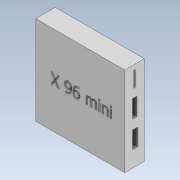
# Autodesk Inventor part: Медиа приставка GIBORIY X96 Mini 2
Saved by Autodesk Inventor 2021.2 (Build 252289000, 289)
## iProperties
Created: 2022-11-29
Part Number: Медиа приставка GIBORIY X96 Mini 2
Material: Типовые
Document SubType Name: Modeling
Designer: Voodoo
Mass: 114.64 g
Surface Area: 238.678 cm^2
Volume: 114.64 cm^3
Density: 1 g/cm^3
Appearance: По умолчанию
Author: Voodoo
Autodesk Inventor part; units mm, degrees
ref_plane "YZ Plane" through (0, 0, 0) normal (1, 0, 0) x (0, 1, 0)
ref_plane "XZ Plane" through (0, 0, 0) normal (0, 1, 0) x (-1, 0, 0)
ref_plane "XY Plane" through (0, 0, 0) normal (0, 0, 1) x (1, 0, 0)
sketch "Эскиз1" plane through (0, 0, 0) normal (0, 0, 1) x (1, 0, 0)
  line L0 (-41, -41) -> (41, -41)
  line L1 (41, -41) -> (41, 41)
  line L2 (41, 41) -> (-41, 41)
  line L3 (-41, 41) -> (-41, -41)
  line L4 (-41, -41) -> (41, 41) construction
  line L5 (41, -41) -> (-41, 41) construction
  point P0 (0, 0)
  dimension "d0" = 82
  dimension "d1" = 82
  constraints: 12 end point, 2 midpoint, 2 parallel, 1 horizontal, 1 perpendicular
  measures "d0" distance of L2.end L1.end
  measures "d1" distance of L1.end L0.end
extrude "Выдавливание1" add sketch "Эскиз1" along normal blind 18
sketch "Эскиз2" plane through (-41, -41, 0) normal (0, -1, 0) x (1, 0, 0)
  line L0 (0, 0) -> (82, 0) projected
  line L1 (82, 0) -> (82, 18) projected
  line L2 (0, 18) -> (82, 18) projected
  line L3 (0, 0) -> (0, 18) projected
  line L4 (21.3532, 13.2427) -> (31.0848, 13.2427)
  line L5 (31.0848, 13.2427) -> (31.0848, 4.7964)
  line L6 (31.0848, 4.7964) -> (21.3532, 4.7964)
  line L7 (21.3532, 4.7964) -> (21.3532, 13.2427)
  line L8 (39.8983, 10.8557) -> (49.9971, 10.8557)
  line L9 (49.9971, 10.8557) -> (49.9971, 6.6326)
  line L10 (49.9971, 6.6326) -> (39.8983, 6.6326)
  line L11 (39.8983, 6.6326) -> (39.8983, 10.8557)
  circle A0 centre (11.6216, 9.0196) radius 2.5509
  circle A1 centre (62.1157, 9.0196) radius 2.4635
  circle A2 centre (73.6834, 9.0196) radius 2.6481
  point P0 (41, 0)
  constraints: 16 end point, 4 parallel, 3 centre point, 2 horizontal, 2 perpendicular
extrude "Выдавливание2" cut sketch "Эскиз2" against normal blind 18 contours L4 L5 L6 L7 | L8 L9 L10 L11 | A0 | A1 | A2
sketch "Эскиз3" plane through (41, -41, 0) normal (1, 0, 0) x (0, 0, -1)
  line L0 (-10.7302, 14.7828) -> (-6.0842, 14.7828)
  line L1 (-6.0842, 14.7828) -> (-6.0842, 30.3804)
  line L2 (-6.0842, 30.3804) -> (-10.7302, 30.3804)
  line L3 (-10.7302, 30.3804) -> (-10.7302, 14.7828)
  line L4 (-10.7302, 39.3407) -> (-6.8585, 39.3407)
  line L5 (-6.8585, 39.3407) -> (-6.8585, 55.4913)
  line L6 (-6.8585, 55.4913) -> (-10.7302, 55.4913)
  line L7 (-10.7302, 55.4913) -> (-10.7302, 39.3407)
  line L8 (-9.7346, 63.3454) -> (-8.4072, 63.3454)
  line L9 (-8.4072, 63.3454) -> (-8.4072, 77.6155)
  line L10 (-8.4072, 77.6155) -> (-9.7346, 77.6155)
  line L11 (-9.7346, 77.6155) -> (-9.7346, 63.3454)
  point P0 (0, 41)
  constraints: 24 end point, 6 parallel, 3 horizontal, 3 perpendicular, 1 point on line
extrude "Выдавливание3" cut sketch "Эскиз3" against normal blind 18
sketch "Эскиз4" plane through (0, 0, 18) normal (0, 0, 1) x (1, 0, 0)
  line L0 (-27.0223, 6.153) -> (33.3984, 6.153) construction
  line L1 (33.3984, 6.153) -> (33.3984, -5.3882) construction
  line L2 (33.3984, -5.3882) -> (-27.0223, -5.3882) construction
  line L3 (-27.0223, -5.3882) -> (-27.0223, 6.153) construction
  line L4 (-19.0969, -4.0496) -> (-20.6204, -4.0496)
  line L5 (-20.6204, -4.0496) -> (-23.0515, -0.0626)
  line L6 (-23.0515, -0.0626) -> (-25.5312, -4.0496)
  line L7 (-25.5312, -4.0496) -> (-26.9656, -4.0496)
  line L8 (-26.9656, -4.0496) -> (-23.7808, 0.9585)
  line L9 (-23.7808, 0.9585) -> (-26.8683, 5.9504)
  line L10 (-26.8683, 5.9504) -> (-25.3448, 5.9504)
  line L11 (-25.3448, 5.9504) -> (-22.9623, 2.0363)
  line L12 (-22.9623, 2.0363) -> (-20.5312, 5.9504)
  line L13 (-20.5312, 5.9504) -> (-19.0969, 5.9504)
  line L14 (-19.0969, 5.9504) -> (-22.2249, 1.0233)
  line L15 (-22.2249, 1.0233) -> (-19.0969, -4.0496)
  spline S0 degree 2 poles (-14.2913, 2.7008) (-14.2913, 3.4707) (-13.7889, 4.751) (-13.3513, 5.213) knots 0 0 0 1 2 2 2
  spline S1 degree 2 poles (-13.3513, 5.213) (-12.938, 5.6587) (-11.7306, 6.153) (-11.1147, 6.153) knots 0 0 0 1 2 2 2
  spline S2 degree 2 poles (-11.1147, 6.153) (-10.4259, 6.153) (-9.3076, 5.6911) (-8.8943, 5.2535) knots 0 0 0 1 2 2 2
  spline S3 degree 2 poles (-8.8943, 5.2535) (-8.3756, 4.7024) (-7.8084, 2.9196) (-7.8084, 1.5501) knots 0 0 0 1 2 2 2
  spline S4 degree 2 poles (-7.8084, 1.5501) (-7.8084, 0.3102) (-8.3675, -1.9102) (-8.9105, -2.6477) knots 0 0 0 1 2 2 2
  spline S5 degree 2 poles (-8.9105, -2.6477) (-9.4858, -3.4256) (-11.1066, -4.2441) (-12.2897, -4.2441) knots 0 0 0 1 2 2 2
  spline S6 degree 2 poles (-12.2897, -4.2441) (-12.5571, -4.2441) (-13.1649, -4.1874) (-13.4242, -4.1063) knots 0 0 0 1 2 2 2
  line L16 (-13.4242, -4.1063) -> (-13.4242, -2.8178)
  line L17 (-13.4242, -2.8178) -> (-13.3594, -2.8178)
  spline S7 degree 2 poles (-13.3594, -2.8178) (-13.1892, -2.9151) (-12.4761, -3.0853) (-12.1114, -3.0853) knots 0 0 0 1 2 2 2
  spline S8 degree 2 poles (-12.1114, -3.0853) (-10.7986, -3.0853) (-9.2994, -1.3511) (-9.1941, 0.2535) knots 0 0 0 1 2 2 2
  spline S9 degree 2 poles (-9.1941, 0.2535) (-9.7289, -0.1112) (-10.7014, -0.4434) (-11.2768, -0.4434) knots 0 0 0 1 2 2 2
  spline S10 degree 2 poles (-11.2768, -0.4434) (-11.8278, -0.4434) (-12.7435, -0.2003) (-13.2054, 0.1481) knots 0 0 0 1 2 2 2
  spline S11 degree 2 poles (-13.2054, 0.1481) (-13.7403, 0.5614) (-14.2913, 1.8175) (-14.2913, 2.7008) knots 0 0 0 1 2 2 2
  spline S12 degree 2 poles (-9.1617, 1.8499) (-9.1617, 2.8629) (-9.5345, 4.1433) (-9.8667, 4.4917) knots 0 0 0 1 2 2 2
  spline S13 degree 2 poles (-9.8667, 4.4917) (-10.1584, 4.8159) (-10.7662, 5.059) (-11.1228, 5.059) knots 0 0 0 1 2 2 2
  spline S14 degree 2 poles (-11.1228, 5.059) (-11.9494, 5.059) (-12.9299, 3.8758) (-12.9299, 2.7575) knots 0 0 0 1 2 2 2
  spline S15 degree 2 poles (-12.9299, 2.7575) (-12.9299, 2.1254) (-12.6058, 1.307) (-12.2492, 1.0152) knots 0 0 0 1 2 2 2
  spline S16 degree 2 poles (-12.2492, 1.0152) (-11.9899, 0.8045) (-11.3497, 0.6668) (-10.9769, 0.6668) knots 0 0 0 1 2 2 2
  spline S17 degree 2 poles (-10.9769, 0.6668) (-10.5474, 0.6668) (-9.5588, 0.9666) (-9.186, 1.2178) knots 0 0 0 1 2 2 2
  spline S18 degree 2 poles (-9.186, 1.2178) (-9.1779, 1.3151) (-9.1617, 1.6473) (-9.1617, 1.8499) knots 0 0 0 1 2 2 2
  spline S19 degree 2 poles (-0.1909, -0.8081) (-0.1909, -1.578) (-0.7014, -2.8827) (-1.1309, -3.3203) knots 0 0 0 1 2 2 2
  spline S20 degree 2 poles (-1.1309, -3.3203) (-1.5766, -3.7822) (-2.6949, -4.2603) (-3.3675, -4.2603) knots 0 0 0 1 2 2 2
  spline S21 degree 2 poles (-3.3675, -4.2603) (-4.0401, -4.2603) (-5.1503, -3.8065) (-5.5717, -3.3527) knots 0 0 0 1 2 2 2
  spline S22 degree 2 poles (-5.5717, -3.3527) (-6.0904, -2.8097) (-6.6738, -0.9864) (-6.6738, 0.3426) knots 0 0 0 1 2 2 2
  spline S23 degree 2 poles (-6.6738, 0.3426) (-6.6738, 1.6473) (-6.139, 3.7462) (-5.5798, 4.5241) knots 0 0 0 1 2 2 2
  spline S24 degree 2 poles (-5.5798, 4.5241) (-5.0369, 5.2859) (-3.3189, 6.1368) (-2.1925, 6.1368) knots 0 0 0 1 2 2 2
  spline S25 degree 2 poles (-2.1925, 6.1368) (-1.8602, 6.1368) (-1.2768, 6.072) (-1.058, 5.999) knots 0 0 0 1 2 2 2
  line L18 (-1.058, 5.999) -> (-1.058, 4.7105)
  line L19 (-1.058, 4.7105) -> (-1.1147, 4.7105)
  spline S26 degree 2 poles (-1.1147, 4.7105) (-1.3011, 4.8078) (-1.9818, 4.978) (-2.3708, 4.978) knots 0 0 0 1 2 2 2
  spline S27 degree 2 poles (-2.3708, 4.978) (-3.6187, 4.978) (-5.1503, 3.2924) (-5.2962, 1.6392) knots 0 0 0 1 2 2 2
  spline S28 degree 2 poles (-5.2962, 1.6392) (-4.8181, 1.9715) (-3.8132, 2.3361) (-3.2135, 2.3361) knots 0 0 0 1 2 2 2
  spline S29 degree 2 poles (-3.2135, 2.3361) (-2.6301, 2.3361) (-1.7549, 2.1011) (-1.2768, 1.7446) knots 0 0 0 1 2 2 2
  spline S30 degree 2 poles (-1.2768, 1.7446) (-0.7257, 1.3313) (-0.1909, 0.0509) (-0.1909, -0.8081) knots 0 0 0 1 2 2 2
  spline S31 degree 2 poles (-1.5523, -0.8648) (-1.5523, -0.249) (-1.8764, 0.5857) (-2.233, 0.8775) knots 0 0 0 1 2 2 2
  spline S32 degree 2 poles (-2.233, 0.8775) (-2.5004, 1.0882) (-3.1649, 1.2259) (-3.5134, 1.2259) knots 0 0 0 1 2 2 2
  spline S33 degree 2 poles (-3.5134, 1.2259) (-3.9834, 1.2259) (-4.8667, 0.9423) (-5.2962, 0.6749) knots 0 0 0 1 2 2 2
  spline S34 degree 2 poles (-5.2962, 0.6749) (-5.3043, 0.529) (-5.3205, 0.2535) (-5.3205, 0.0428) knots 0 0 0 1 2 2 2
  spline S35 degree 2 poles (-5.3205, 0.0428) (-5.3205, -0.9945) (-4.9153, -2.2668) (-4.6074, -2.599) knots 0 0 0 1 2 2 2
  spline S36 degree 2 poles (-4.6074, -2.599) (-4.3238, -2.9151) (-3.7079, -3.1663) (-3.3594, -3.1663) knots 0 0 0 1 2 2 2
  spline S37 degree 2 poles (-3.3594, -3.1663) (-2.549, -3.1663) (-1.5523, -2.0156) (-1.5523, -0.8648) knots 0 0 0 1 2 2 2
  line L20 (13.9826, -4.0496) -> (13.9826, 0.294)
  spline S38 degree 2 poles (13.9826, 0.294) (13.9826, 0.8126) (13.9015, 1.6959) (13.7719, 1.9391) knots 0 0 0 1 2 2 2
  spline S39 degree 2 poles (13.7719, 1.9391) (13.6422, 2.2065) (13.1479, 2.4658) (12.7184, 2.4658) knots 0 0 0 1 2 2 2
  spline S40 degree 2 poles (12.7184, 2.4658) (12.3294, 2.4658) (11.438, 1.9877) (10.968, 1.5339) knots 0 0 0 1 2 2 2
  spline S41 degree 2 poles (10.968, 1.5339) (10.9761, 1.4204) (10.9923, 1.1044) (10.9923, 0.8937) knots 0 0 0 1 2 2 2
  line L21 (10.9923, 0.8937) -> (10.9923, -4.0496)
  line L22 (10.9923, -4.0496) -> (9.7281, -4.0496)
  line L23 (9.7281, -4.0496) -> (9.7281, 0.294)
  spline S42 degree 2 poles (9.7281, 0.294) (9.7281, 0.8126) (9.6471, 1.6959) (9.5174, 1.9391) knots 0 0 0 1 2 2 2
  spline S43 degree 2 poles (9.5174, 1.9391) (9.3877, 2.2065) (8.8934, 2.4658) (8.4639, 2.4658) knots 0 0 0 1 2 2 2
  spline S44 degree 2 poles (8.4639, 2.4658) (8.0587, 2.4658) (7.1592, 1.9553) (6.7378, 1.5582) knots 0 0 0 1 2 2 2
  line L24 (6.7378, 1.5582) -> (6.7378, -4.0496)
  line L25 (6.7378, -4.0496) -> (5.4736, -4.0496)
  line L26 (5.4736, -4.0496) -> (5.4736, 3.4545)
  line L27 (5.4736, 3.4545) -> (6.7378, 3.4545)
  line L28 (6.7378, 3.4545) -> (6.7378, 2.6279)
  spline S45 degree 2 poles (6.7378, 2.6279) (7.2322, 3.1222) (8.2046, 3.6651) (8.7881, 3.6651) knots 0 0 0 1 2 2 2
  spline S46 degree 2 poles (8.7881, 3.6651) (9.4526, 3.6651) (10.4818, 3.0574) (10.7492, 2.3686) knots 0 0 0 1 2 2 2
  spline S47 degree 2 poles (10.7492, 2.3686) (11.3245, 3.0087) (12.4104, 3.6651) (13.0425, 3.6651) knots 0 0 0 1 2 2 2
  spline S48 degree 2 poles (13.0425, 3.6651) (13.5288, 3.6651) (14.3229, 3.3653) (14.6147, 3.025) knots 0 0 0 1 2 2 2
  spline S49 degree 2 poles (14.6147, 3.025) (14.9145, 2.6846) (15.2467, 1.6635) (15.2467, 0.8937) knots 0 0 0 1 2 2 2
  line L29 (15.2467, 0.8937) -> (15.2467, -4.0496)
  line L30 (15.2467, -4.0496) -> (13.9826, -4.0496)
  line L31 (18.31, -4.0496) -> (17.0458, -4.0496)
  line L32 (17.0458, -4.0496) -> (17.0458, 3.4545)
  line L33 (17.0458, 3.4545) -> (18.31, 3.4545)
  line L34 (18.31, 3.4545) -> (18.31, -4.0496)
  line L35 (18.3991, 4.7024) -> (16.9647, 4.7024)
  line L36 (16.9647, 4.7024) -> (16.9647, 6.0152)
  line L37 (16.9647, 6.0152) -> (18.3991, 6.0152)
  line L38 (18.3991, 6.0152) -> (18.3991, 4.7024)
  line L39 (26.0571, -4.0496) -> (24.7929, -4.0496)
  line L40 (24.7929, -4.0496) -> (24.7929, 0.2292)
  spline S50 degree 2 poles (24.7929, 0.2292) (24.7929, 0.7478) (24.6957, 1.6392) (24.5498, 1.9066) knots 0 0 0 1 2 2 2
  spline S51 degree 2 poles (24.5498, 1.9066) (24.3959, 2.1903) (23.8448, 2.4658) (23.3748, 2.4658) knots 0 0 0 1 2 2 2
  spline S52 degree 2 poles (23.3748, 2.4658) (22.9048, 2.4658) (21.908, 1.9634) (21.4299, 1.5582) knots 0 0 0 1 2 2 2
  line L41 (21.4299, 1.5582) -> (21.4299, -4.0496)
  line L42 (21.4299, -4.0496) -> (20.1657, -4.0496)
  line L43 (20.1657, -4.0496) -> (20.1657, 3.4545)
  line L44 (20.1657, 3.4545) -> (21.4299, 3.4545)
  line L45 (21.4299, 3.4545) -> (21.4299, 2.6198)
  spline S53 degree 2 poles (21.4299, 2.6198) (21.9971, 3.1303) (23.0912, 3.6651) (23.707, 3.6651) knots 0 0 0 1 2 2 2
  spline S54 degree 2 poles (23.707, 3.6651) (24.8091, 3.6651) (26.0571, 2.2065) (26.0571, 0.8207) knots 0 0 0 1 2 2 2
  line L46 (26.0571, 0.8207) -> (26.0571, -4.0496)
  line L47 (29.1203, -4.0496) -> (27.8561, -4.0496)
  line L48 (27.8561, -4.0496) -> (27.8561, 3.4545)
  line L49 (27.8561, 3.4545) -> (29.1203, 3.4545)
  line L50 (29.1203, 3.4545) -> (29.1203, -4.0496)
  line L51 (29.2095, 4.7024) -> (27.7751, 4.7024)
  line L52 (27.7751, 4.7024) -> (27.7751, 6.0152)
  line L53 (27.7751, 6.0152) -> (29.2095, 6.0152)
  line L54 (29.2095, 6.0152) -> (29.2095, 4.7024)
  point P0 (0, 0)
  constraints: 2 other
extrude "Выдавливание4" cut sketch "Эскиз4" against normal blind 2
